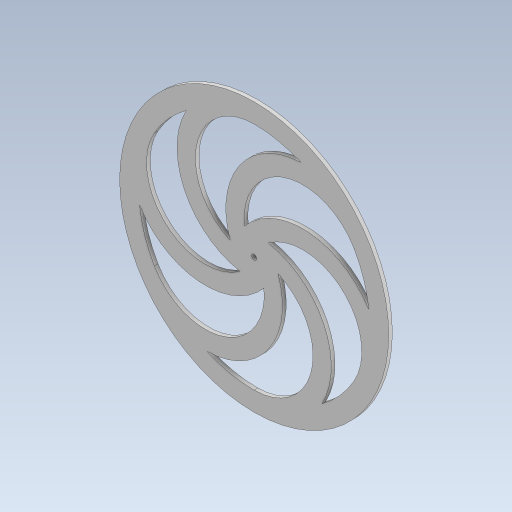
# Autodesk Inventor part: gear backing end
Saved by Autodesk Inventor 2023 (Build 270158000, 158)
## iProperties
Created: 2023-03-22
Part Number: gear backing end
Material: Generic
Document SubType Name: Modeling
Designer: dverd
Density: 1 g/cm^3
Appearance: Default
Author: dverd
Autodesk Inventor part; units mm, degrees
ref_plane "YZ Plane" through (0, 0, 0) normal (1, 0, 0) x (0, 1, 0)
ref_plane "XZ Plane" through (0, 0, 0) normal (0, 1, 0) x (-1, 0, 0)
ref_plane "XY Plane" through (0, 0, 0) normal (0, 0, 1) x (1, 0, 0)
sketch "Sketch1" plane through (0, 0, 0) normal (0, 0, 1) x (1, 0, 0)
  circle A0 centre (0, 0) radius 93.4212
  dimension "d0" = 186.8424
  constraints: 1 centre point, 1 coincident
  measures "d0" diameter of A0
extrude "Extrusion1" add sketch "Sketch1" along normal blind 2.54
sketch "Sketch2" plane through (0, 0, 2.54) normal (0, 0, 1) x (1, 0, 0)
  circle A0 centre (0, 0) radius 1.75
  circle A1 centre (0, 0) radius 14.45
  circle A2 centre (0, 0) radius 92.71
  circle A3 centre (0, 0) radius 80.01
  arc A4 (0, -80.01) -> (0, 1.75) centre (0, -39.13) ccw
  arc A5 (0, -92.71) -> (0, 14.45) centre (0, -39.13) ccw
  arc A6 (80.2892, -46.355) -> (-12.5141, 7.225) centre (33.8876, -19.565) ccw
  arc A7 (69.2907, -40.005) -> (-1.5155, 0.875) centre (33.8876, -19.565) ccw
  arc A8 (80.2892, 46.355) -> (-12.5141, -7.225) centre (33.8876, 19.565) ccw
  arc A9 (69.2907, 40.005) -> (-1.5155, -0.875) centre (33.8876, 19.565) ccw
  arc A10 (0, 92.71) -> (0, -14.45) centre (0, 39.13) ccw
  arc A11 (0, 80.01) -> (0, -1.75) centre (0, 39.13) ccw
  arc A12 (-80.2892, 46.355) -> (12.5141, -7.225) centre (-33.8876, 19.565) ccw
  arc A13 (-69.2907, 40.005) -> (1.5155, -0.875) centre (-33.8876, 19.565) ccw
  arc A14 (-80.2892, -46.355) -> (12.5141, 7.225) centre (-33.8876, -19.565) ccw
  arc A15 (-69.2907, -40.005) -> (1.5155, 0.875) centre (-33.8876, -19.565) ccw
  point P0 (-69.2907, -40.005)
  point P1 (6.7724, -15.3289)
  point P2 (-79.5631, -8.4451)
  point P3 (16.6614, -1.7994)
  point P4 (-32.4678, -73.1262)
  point P5 (9.8891, 13.5295)
  point P6 (47.0952, -64.6811)
  point P7 (69.2907, 40.005)
  point P8 (-6.7724, 15.3289)
  point P9 (79.5631, 8.4451)
  point P10 (0, 80.01)
  point P11 (-16.6614, 1.7994)
  point P12 (32.4678, 73.1262)
  point P13 (-9.8891, -13.5295)
  point P14 (-47.0952, 64.6811)
  dimension "d3" = 3.5
  dimension "d15" = 12.7
  dimension "d17" = 185.42
  dimension "d18" = 160.02
  dimension "d21" = 360
  constraints: 24 point on circle, 12 centre point, 3 vertical alignment, 2 coincident, 62 other
extrude "Extrusion2" cut sketch "Sketch2" against normal blind 2.54 contours A0 | A15 A3 A12 | A13 A3 A10 | A4 A3 A14 | A11 A3 A8 | A7 A3 A5 | A9 A3 A6
body "Solid1"
